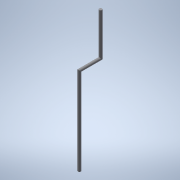
# Autodesk Inventor part: 00_Beam_Stairs_7.5mm
Saved by Autodesk Inventor 2022 (Build 260153000, 153)
## iProperties
Created: 2021-11-23
Part Number: 00_Beam_Stairs_7.5mm
Material: Generisch
Document SubType Name: Modeling
Designer: UC2
Density: 1 g/cm^3
Appearance: Vorgabe
Author: UC2
Autodesk Inventor part; units mm, degrees
ref_plane "YZ Plane" through (0, 0, 0) normal (1, 0, 0) x (0, 1, 0)
ref_plane "XZ Plane" through (0, 0, 0) normal (0, 1, 0) x (-1, 0, 0)
ref_plane "XY Plane" through (0, 0, 0) normal (0, 0, 1) x (1, 0, 0)
sketch "Skizze1" plane through (0, 0, 0) normal (1, 0, 0) x (0, 1, 0)
  line L0 (0, 0) -> (-15, 0)
  line L1 (-15, 0) -> (-15, 7.5)
  line L2 (-15, 7.5) -> (-45.667, 7.5)
  dimension "d0" = 15
  dimension "d1" = 7.5
  constraints: 6 end point, 2 perpendicular, 1 horizontal
  measures "d0" distance of L0.start L0.end
  measures "d1" distance of L0.end L1.end
sketch "Skizze2" plane through (0, 0, 0) normal (0, 1, 0) x (-1, 0, 0)
  circle A0 centre (0, 0) radius 0.5
  dimension "d2" = 1
  constraints: 1 centre point, 1 coincident
  measures "d2" diameter of A0
sweep "Sweeping1" add profiles "Skizze2" path "Skizze1"
sketch "Skizze3" plane through (0, 0, 0) normal (1, 0, 0) x (0, 1, 0)
  line L0 (-14.5, 0.5) -> (-14.5, 8) projected
  line L1 (-15.5, -0.5) -> (-15.5, 7) projected
  line L2 (-13.783, 17.8624) -> (-5.8155, 9.8948)
  line L3 (-5.8155, 9.8948) -> (-11.6052, 4.1052)
  line L4 (-11.6052, 4.1052) -> (-19.5727, 12.0727)
  line L5 (-19.5727, 12.0727) -> (-13.783, 17.8624)
  line L6 (-13.783, 17.8624) -> (-11.6052, 4.1052) construction
  line L7 (-5.8155, 9.8948) -> (-19.5727, 12.0727) construction
  line L8 (-13.783, 17.8624) -> (-2.5152, 17.8624) construction
  line L9 (-14.4975, -10.7606) -> (-21.8094, -3.4488)
  line L10 (-21.8094, -3.4488) -> (-16.6803, 1.6803)
  line L11 (-16.6803, 1.6803) -> (-9.3684, -5.6316)
  line L12 (-9.3684, -5.6316) -> (-14.4975, -10.7606)
  line L13 (-14.4975, -10.7606) -> (-16.6803, 1.6803) construction
  line L14 (-21.8094, -3.4488) -> (-9.3684, -5.6316) construction
  point P0 (0, 0)
  point P1 (-12.6941, 10.9838)
  point P2 (-15.5889, -4.5402)
  dimension "d5" = 45
  constraints: 26 end point, 4 midpoint, 4 parallel, 3 perpendicular, 1 equal length, 1 horizontal
  measures "d5" angle of L2 L8
extrude "Extrusion1" cut sketch "Skizze3" along normal through all both and the other way through all
